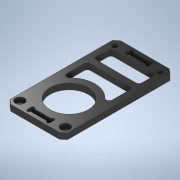
# Autodesk Inventor part: Trunk_neck_frame
Saved by Autodesk Inventor 2022 (Build 260153000, 153)
## iProperties
Part Number: Trunk_neck_frame
Material: アルミニウム 2014-T4
Document SubType Name: Modeling
Designer: Masato Kubotera
Density: 2.8 g/cm^3
Appearance: 光沢 - 黒
Mass: 15.4453 g
Surface Area: 52.3593 cm^2
Volume: 5.51618 cm^3
Description: A2017 T4
Author: Masato Kubotera
Autodesk Inventor part; units mm, degrees
ref_plane "YZ Plane" through (0, 0, 0) normal (1, 0, 0) x (0, 1, 0)
ref_plane "XZ Plane" through (0, 0, 0) normal (0, 1, 0) x (-1, 0, 0)
ref_plane "XY Plane" through (0, 0, 0) normal (0, 0, 1) x (1, 0, 0)
sketch "スケッチ1" plane through (0, 0, 0) normal (0, 0, 1) x (1, 0, 0)
  circle A0 centre (0, 0) radius 10.5 construction
  line L0 (-28, -13.5) -> (-1, -13.5) construction
  line L1 (-1, -13.5) -> (-1, 13.5) construction
  line L2 (-1, 13.5) -> (-28, 13.5) construction
  line L3 (-28, 13.5) -> (-28, -13.5) construction
  line L4 (-28, -13.5) -> (-1, 13.5) construction
  line L5 (-1, -13.5) -> (-28, 13.5) construction
  line L6 (-31, -16) -> (12, -16) construction
  line L7 (12, -16) -> (12, 16) construction
  line L8 (12, 16) -> (-31, 16) construction
  line L9 (-31, 16) -> (-31, -16) construction
  line L10 (-31, -16) -> (12, 16) construction
  line L11 (12, -16) -> (-31, 16) construction
  line L12 (-31, -14.4) -> (-39.5, -14.4) construction
  line L13 (-39.5, -14.4) -> (-39.5, 14.4) construction
  line L14 (-39.5, 0) -> (12, 0) construction
  line L15 (-31, 14.4) -> (-39.5, 14.4) construction
  line L16 (-14.5, -13.5) -> (-14.5, 13.5) construction
  line L17 (17.5, -7.5) -> (20, -7.5) construction
  line L18 (20, -7.5) -> (20, 7.5) construction
  line L19 (20, 7.5) -> (17.5, 7.5) construction
  line L20 (17.5, 7.5) -> (17.5, -7.5) construction
  line L21 (17.5, -7.5) -> (20, 7.5) construction
  line L22 (20, -7.5) -> (17.5, 7.5) construction
  line L23 (17.45, 7.55) -> (20.05, 7.55)
  line L24 (20.05, 5.45) -> (20.05, -5.45)
  line L25 (20.05, -7.55) -> (17.45, -7.55)
  line L26 (17.45, -5.45) -> (17.45, 5.45)
  line L27 (17.45, 7.55) -> (20.05, -7.55) construction
  line L28 (20.05, 7.55) -> (17.45, -7.55) construction
  arc A1 (17.45, -5.45) -> (17.45, -7.55) centre (17.45, -6.5) ccw
  line L29 (18.75, -7.5) -> (18.75, 7.5) construction
  arc A2 (17.45, 7.55) -> (17.45, 5.45) centre (17.45, 6.5) ccw
  arc A3 (20.05, -7.55) -> (20.05, -5.45) centre (20.05, -6.5) ccw
  arc A4 (20.05, 5.45) -> (20.05, 7.55) centre (20.05, 6.5) ccw
  line L30 (-13.75, -16) -> (-13.75, 16) construction
  line L31 (-45, -7.5) -> (-47.5, -7.5) construction
  line L32 (-47.5, -7.5) -> (-47.5, 7.5) construction
  line L33 (-47.5, 7.5) -> (-45, 7.5) construction
  line L34 (-45, 7.5) -> (-45, -7.5) construction
  line L35 (-45, -7.5) -> (-47.5, 7.5) construction
  line L36 (-47.5, -7.5) -> (-45, 7.5) construction
  line L37 (-44.95, 7.55) -> (-47.55, 7.55)
  line L38 (-47.55, 5.45) -> (-47.55, -5.45)
  line L39 (-47.55, -7.55) -> (-44.95, -7.55)
  line L40 (-44.95, -5.45) -> (-44.95, 5.45)
  line L41 (-44.95, 7.55) -> (-47.55, -7.55) construction
  line L42 (-47.55, 7.55) -> (-44.95, -7.55) construction
  arc A5 (-44.95, -7.55) -> (-44.95, -5.45) centre (-44.95, -6.5) ccw
  line L43 (-46.25, -7.5) -> (-46.25, 7.5) construction
  arc A6 (-44.95, 5.45) -> (-44.95, 7.55) centre (-44.95, 6.5) ccw
  arc A7 (-47.55, -5.45) -> (-47.55, -7.55) centre (-47.55, -6.5) ccw
  arc A8 (-47.55, 7.55) -> (-47.55, 5.45) centre (-47.55, 6.5) ccw
  circle A9 centre (17.5, -15) radius 1.6
  circle A10 centre (17.5, 15) radius 1.6
  circle A11 centre (-45, -15) radius 1.6
  circle A12 centre (-45, 15) radius 1.6
  line L44 (15, -60.5) -> (20, -60.5) construction
  line L45 (20, -60.5) -> (20, 60.5) construction
  line L46 (20, 60.5) -> (15, 60.5) construction
  line L47 (15, -60.5) -> (20, 60.5) construction
  line L48 (20, -60.5) -> (15, 60.5) construction
  arc A13 (-6.5678, 15) -> (-6.5678, -15) centre (-1, 0) ccw
  line L49 (-3.65, -16) -> (1.65, -16) construction
  line L50 (1.65, -16) -> (1.65, 16) construction
  line L51 (1.65, 16) -> (-3.65, 16) construction
  line L52 (-3.65, 16) -> (-3.65, -16) construction
  line L53 (-3.65, -16) -> (1.65, 16) construction
  line L54 (1.65, -16) -> (-3.65, 16) construction
  line L55 (-42.5, -60.5) -> (-47.5, -60.5) construction
  line L56 (-47.5, -60.5) -> (-47.5, 60.5) construction
  line L57 (-47.5, 60.5) -> (-42.5, 60.5) construction
  line L58 (-42.5, 60.5) -> (-42.5, -60.5) construction
  circle A14 centre (17.5, -15) radius 3
  circle A15 centre (17.5, 15) radius 3
  line L59 (-27, -15) -> (-6.5678, -15)
  line L60 (-42.5, -15) -> (-31, -15)
  line L61 (-31, -15) -> (-31, 15)
  line L62 (-31, 15) -> (-42.5, 15)
  line L63 (-42.5, 15) -> (-42.5, -15)
  line L64 (-42.5, -15) -> (-31, 15) construction
  line L65 (-31, -15) -> (-42.5, 15) construction
  line L66 (-47.5, -19) -> (20, -19)
  line L67 (-27, -15) -> (-27, 15)
  line L68 (-47.5, 19) -> (20, 19)
  line L69 (20, -19) -> (22.5, -16.0779)
  line L70 (22.5, -16.0779) -> (22.5, 16.0779)
  line L71 (20, 19) -> (22.5, 16.0779)
  line L72 (-47.5, -19) -> (-50, -16.0779)
  line L73 (-50, -16.0779) -> (-50, 16.0779)
  line L74 (-47.5, 19) -> (-50, 16.0779)
  line L75 (-27, 15) -> (-6.5678, 15)
  line L76 (15, 60.5) -> (15, -60.5) construction
  circle A16 centre (0, 0) radius 12.65
  point P0 (-14.5, 0)
  point P1 (-9.5, 0)
  point P2 (-14.5, 0)
  point P3 (18.75, 0)
  point P4 (18.75, 0)
  point P5 (18.75, 0)
  point P6 (18.75, 0)
  point P7 (-46.25, 0)
  point P8 (-46.25, 0)
  point P9 (-46.25, 0)
  point P10 (-46.25, 0)
  point P11 (17.5, 0)
  point P12 (17.5, 0)
  point P13 (-1, 0)
  point P14 (-36.75, 0)
  point P15 (-1, 0)
  dimension "d0" = 21
  dimension "d1" = 27
  dimension "d2" = 27
  dimension "d3" = 43
  dimension "d4" = 32
  dimension "d5" = 28.8
  dimension "d6" = 8.5
  dimension "d7" = 9.5
  dimension "d11" = 8.5
  dimension "d13" = 2.5
  dimension "d14" = 15
  dimension "d15" = 1.05
  dimension "d16" = 0.05
  dimension "d17" = 0.05
  dimension "d28" = 3.2
  dimension "d31" = 5
  dimension "d32" = 121
  dimension "d36" = 5.3
  dimension "d55" = 16
  dimension "d71" = 6
  dimension "d83" = 30
  dimension "d84" = 2.5
  dimension "d97" = 1.5
  dimension "d98" = 2.5
  dimension "d102" = 38
  dimension "d103" = 4
  dimension "d104" = 4
  dimension "d106" = 2.5
  dimension "d107" = 2.5
  dimension "d108" = 3
  dimension "d109" = 57.5
  dimension "d113" = 25.3
  constraints: 152 end point, 34 symmetric about line, 32 midpoint, 18 point on circle, 17 centre point, 15 parallel, 11 perpendicular, 10 vertical alignment, 8 point on line, 7 horizontal, 4 coincident, 3 equal radius, 2 collinear, 2 vertical, 1 tangent, 18 other
  measures "d0" diameter of A0
  measures "d1" distance of L2.end L1.end
  measures "d2" distance of L1.end L0.end
  measures "d3" distance of L8.end L7.end
  measures "d4" distance of L7.end L6.end
  measures "d5" distance of L12.end L13.end
  measures "d6" distance of L12.start L12.end
  measures "d7" distance of point (0, 0) point (-9.5, 0)
  measures "d11" distance from line of L1 point (-9.5, 0)
  measures "d13" distance of L19.end L18.end
  measures "d14" distance of L18.end L17.end
  measures "d15" radius of A1
  measures "d16" distance between parallel lines of L26 L20
  measures "d17" distance between parallel lines of L25 L17
  measures "d28" diameter of A9
  measures "d31" distance of L46.end L45.end
  measures "d32" distance of L45.end L44.end
  measures "d36" distance of L51.end L50.end
  measures "d55" radius of A13
  measures "d71" diameter of A14
  measures "d83" distance of A10.centre A9.centre
  measures "d84" distance between parallel lines of L63 L34
  measures "d97" distance edge to line of A14 L69
  measures "d98" distance between parallel lines of L70 L45
  measures "d102" distance of L68.end L66.end
  measures "d103" distance between parallel lines of L66 L59
  measures "d104" distance between parallel lines of L67 L61
  measures "d106" distance between parallel lines of L70 L18
  measures "d107" distance from line of A9.centre L45
  measures "d108" distance from line of L76 L7.end
  measures "d109" distance of L44.start L58.end
  measures "d113" diameter of A16
extrude "押し出し1" add sketch "スケッチ1" along normal blind 4 contours L72 L73 L74 L68 L71 L70 L69 L66
extrude "押し出し3" add sketch "スケッチ1" along normal blind 0.9 contours A14 | A15
fillet "フィレット1" radius 2 8 edges at (-31, -15, 2) (-42.5, -15, 2) (-42.5, 15, 2) (-31, 15, 2) (-6.5678, -15, 2) (-6.5678, 15, 2) (-27, 15, 2) (-27, -15, 2)
equation "\"d17\" = d16"
